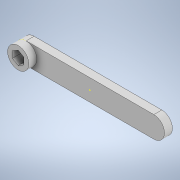
# Autodesk Inventor part: part
Saved by Autodesk Inventor 2020.2 (Build 242310000, 310)
## iProperties
Created: 2020-02-14
Part Number: part
Material: Generic
Document SubType Name: Modeling
Designer: robst
Density: 1 g/cm^3
Appearance: Default
Author: robst
Autodesk Inventor part; units mm, degrees
ref_plane "YZ Plane" through (0, 0, 0) normal (1, 0, 0) x (0, 1, 0)
ref_plane "XZ Plane" through (0, 0, 0) normal (0, 1, 0) x (-1, 0, 0)
ref_plane "XY Plane" through (0, 0, 0) normal (0, 0, 1) x (1, 0, 0)
sketch "Sketch1" plane through (0, 0, 0) normal (0, 0, 1) x (1, 0, 0)
  line L0 (-88.9, -12.7) -> (88.9, -12.7)
  line L1 (88.9, -12.7) -> (88.9, 12.7)
  line L2 (88.9, 12.7) -> (-88.9, 12.7)
  line L3 (-88.9, 12.7) -> (-88.9, -12.7)
  line L4 (-88.9, -12.7) -> (88.9, 12.7) construction
  line L5 (88.9, -12.7) -> (-88.9, 12.7) construction
  point P0 (0, 0)
  dimension "d0" = 177.8
  dimension "d1" = 25.4
  constraints: 12 end point, 2 midpoint, 2 parallel, 1 horizontal, 1 perpendicular
  measures "d0" distance of L2.end L1.end
  measures "d1" distance of L0.end L1.end
extrude "Extrusion1" add sketch "Sketch1" along normal blind 9.525
fillet "Fillet1" radius 12.7 4 edges at (88.9, 12.7, 4.7625) (88.9, -12.7, 4.7625) (-88.9, 12.7, 4.7625) (-88.9, -12.7, 4.7625)
sketch "Sketch2" plane through (0, 0, 9.525) normal (0, 0, 1) x (1, 0, 0)
  arc A0 (-76.2, 12.7) -> (-76.2, -12.7) centre (-76.2, 0) ccw construction
  point P0 (0, 0)
sketch "Sketch3" plane through (0, 0, 9.525) normal (0, 0, 1) x (1, 0, 0)
  line L0 (-76.2, 0) -> (-69.342, 0) construction
  line L1 (-69.342, 3.9653) -> (-69.3369, -3.9566)
  line L2 (-69.3369, -3.9566) -> (-76.1949, -7.9219)
  line L3 (-76.1949, -7.9219) -> (-83.058, -3.9653)
  line L4 (-83.058, -3.9653) -> (-83.0631, 3.9566)
  line L5 (-83.0631, 3.9566) -> (-76.2051, 7.9219)
  line L6 (-76.2051, 7.9219) -> (-69.342, 3.9653)
  point P0 (0, 0)
  dimension "d5" = 6.858
  constraints: 14 end point, 1 coincident, 1 horizontal, 13 other
  measures "d5" distance of L0.start L0.end
sketch "Sketch4" plane through (0, 0, 9.525) normal (0, 0, 1) x (1, 0, 0)
  line L0 (76.2, 12.7) -> (-76.2, 12.7) projected
  circle A0 centre (-76.2023, 0) radius 12.7
  point P0 (0, 0)
  constraints: 3 other
extrude "Extrusion2" add sketch "Sketch4" along normal blind 9.525
extrude "Extrusion3" cut sketch "Sketch3" along normal mid plane 25.4
body "Solid1"
